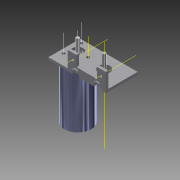
# Autodesk Inventor part: DC motor
Saved by Autodesk Inventor 2013 (Build 170138000, 138)
## iProperties
Created: 2013-01-03
Part Number: DC motor
Material: Generic
Document SubType Name: Modeling
Designer: Nico
Density: 1 g/cm^3
Author: Nico
Autodesk Inventor part; units mm, degrees
ref_plane "YZ Plane" through (0, 0, 0) normal (1, 0, 0) x (0, 1, 0)
ref_plane "XZ Plane" through (0, 0, 0) normal (0, 1, 0) x (-1, 0, 0)
ref_plane "XY Plane" through (0, 0, 0) normal (0, 0, 1) x (1, 0, 0)
sketch "Sketch1" plane through (0, 0, 0) normal (0, 0, 1) x (1, 0, 0)
  line L0 (0, 0) -> (90, 0)
  line L1 (90, 0) -> (90, 50)
  line L2 (90, 50) -> (0, 50)
  line L3 (0, 50) -> (0, 0)
  dimension "d0" = 50
  dimension "d1" = 90
  constraints: 8 end point, 2 parallel, 1 horizontal, 1 perpendicular
  measures "d0" distance of L2.end L0.start
  measures "d1" distance of L0.start L0.end
extrude "Extrusion1" add sketch "Sketch1" along normal blind 4
sketch "Sketch2" plane through (0, 0, 4) normal (0, 0, 1) x (1, 0, 0)
  line L0 (0, 0) -> (90, 0) projected
  line L1 (90, 0) -> (90, 50) projected
  line L2 (0, 50) -> (0, 0) projected
  line L3 (30, 0) -> (90, 0)
  line L4 (90, 0) -> (90, 4)
  line L5 (90, 4) -> (30, 4)
  line L6 (30, 4) -> (30, 0)
  dimension "d4" = 30
  dimension "d5" = 4
  constraints: 8 end point, 2 parallel, 2 point on line, 1 horizontal, 1 perpendicular
  measures "d4" distance between parallel lines of L2 L6
  measures "d5" distance between parallel lines of L0 L5
extrude "Extrusion2" add sketch "Sketch2" along normal blind 25
sketch "Sketch3" plane through (0, 0, 0) normal (0, -1, 0) x (1, 0, 0)
  line L0 (0, 0) -> (90, 0) projected
  line L1 (90, 0) -> (90, 29) projected
  line L2 (30, 29) -> (90, 29) projected
  line L3 (30, 4) -> (30, 29) projected
  line L4 (44, 29) -> (76, 29)
  line L5 (76, 29) -> (76, 12.5)
  line L6 (76, 12.5) -> (44, 12.5)
  line L7 (44, 12.5) -> (44, 29)
  arc A0 (49, 4) -> (37, 4) centre (43, 4) ccw
  line L8 (37, 0) -> (49, 0)
  line L9 (49, 0) -> (49, 4)
  line L10 (37, 4) -> (37, 0)
  line L11 (71, 0) -> (83, 0)
  line L12 (83, 0) -> (83, 4)
  line L13 (71, 4) -> (71, 0)
  arc A1 (83, 4) -> (71, 4) centre (77, 4) ccw
  dimension "d8" = 14
  dimension "d9" = 14
  dimension "d10" = 16.5
  dimension "d11" = 12
  dimension "d13" = 13
  dimension "d14" = 13
  constraints: 20 end point, 4 parallel, 4 point on circle, 3 horizontal, 3 perpendicular, 3 point on line, 2 centre point
  measures "d8" distance between parallel lines of L3 L7
  measures "d9" distance between parallel lines of L5 L1
  measures "d10" distance between parallel lines of L6 L2
  measures "d11" diameter of A0
  measures "d13" distance from line of A0.centre L3
  measures "d14" distance from line of A1.centre L1
extrude "Extrusion3" cut sketch "Sketch3" against normal blind 4
sketch "Sketch4" plane through (0, 0, 0) normal (0, -1, 0) x (1, 0, 0)
  line L0 (76, 29) -> (90, 29) projected
  line L1 (30, 29) -> (44, 29) projected
  line L2 (30, 4) -> (30, 29) projected
  point P0 (38, 19.75)
  point P1 (82, 19.75)
  dimension "d17" = 44
  dimension "d19" = 8
  dimension "d20" = 9.25
  dimension "d21" = 9.25
  measures "d17" distance of point (82, 19.75) point (38, 19.75)
  measures "d19" distance from line of L2 point (38, 19.75)
  measures "d20" distance from line of point (38, 19.75) L1
  measures "d21" distance from line of L0 point (82, 19.75)
hole "Hole1" at (38, 0, 19.75) at (82, 0, 19.75) direction (0, 1, 0) diameter 4.5 end through all
sketch "Sketch5" plane through (0, 0, 4) normal (0, 0, 1) x (1, 0, 0)
  line L0 (90, 50) -> (0, 50) projected
  line L1 (0, 50) -> (0, 0) projected
  circle A0 centre (15, 31) radius 8.5
  circle A1 centre (6.8969, 44.9883) radius 2.25
  circle A2 centre (31.1658, 31.0233) radius 2.25
  circle A3 centre (6.9373, 16.9883) radius 2.25
  dimension "d29" = 19
  dimension "d30" = 15
  dimension "d31" = 17
  dimension "d33" = 4.5
  dimension "d34" = 4.5
  dimension "d35" = 4.5
  constraints: 4 centre point, 1 coincident
  measures "d29" distance from line of A0.centre L0
  measures "d30" distance from line of L1 A0.centre
  measures "d31" diameter of A0
  measures "d33" diameter of A1
  measures "d34" diameter of A2
  measures "d35" diameter of A3
extrude "Extrusion4" cut sketch "Sketch5" against normal blind 4
sketch "Sketch6" plane through (0, 0, 0) normal (0, 0, -1) x (-1, 0, 0)
  circle A0 centre (-6.9373, 16.9883) radius 2.25 projected
  circle A1 centre (-6.8969, 44.9883) radius 2.25 projected
  circle A2 centre (-31.1658, 31.0233) radius 2.25 projected
  circle A3 centre (-6.8969, 44.9883) radius 4
  circle A4 centre (-31.1658, 31.0233) radius 4
  circle A5 centre (-6.9373, 16.9883) radius 4
  dimension "d38" = 8
  dimension "d40" = 8
  dimension "d41" = 8
  constraints: 3 centre point, 3 coincident
  measures "d38" diameter of A4
  measures "d40" diameter of A3
  measures "d41" diameter of A5
extrude "Extrusion5" add sketch "Sketch6" along normal blind 6.35
sketch "Sketch7" plane through (31.1658, 31.0233, -6.35) normal (0, 0, -1) x (-1, 0, 0)
  circle A0 centre (16.1658, 0) radius 21
  line L0 (31.1658, 18.9767) -> (31.1658, -31.0233) projected
  dimension "d44" = 42
  dimension "d47" = 15
  constraints: 1 centre point
  measures "d44" diameter of A0
  measures "d47" distance from line of L0 A0.centre
extrude "Extrusion6" add sketch "Sketch7" along normal blind 85
sketch "Sketch8" plane through (15, 31.0233, -6.35) normal (0, 0, 1) x (1, 0, 0)
  circle A0 centre (0, 0) radius 21 projected
  circle A1 centre (0, 0) radius 8.0116
  point P0 (-15, -31.0233)
  constraints: 1 centre point, 1 coincident
extrude "Extrusion7" add sketch "Sketch8" along normal blind 2 contours A1
sketch "Sketch9" plane through (15, 31.0233, -4.35) normal (0, 0, 1) x (1, 0, 0)
  circle A0 centre (0, 0) radius 8.0116 projected
  circle A1 centre (0, 0) radius 2.5
  point P0 (-15, -31.0233)
  dimension "d52" = 5
  constraints: 1 centre point, 1 coincident
  measures "d52" diameter of A1
extrude "Extrusion8" add sketch "Sketch9" along normal blind 27 contours A1
sketch "Sketch10" plane through (0, 0, 4) normal (0, 0, 1) x (1, 0, 0)
  line L0 (90, 4) -> (90, 50) projected
  line L1 (90, 50) -> (0, 50) projected
  circle A0 centre (60, 27.5) radius 9
  dimension "d56" = 22.5
  dimension "d57" = 30
  dimension "d58" = 18
  constraints: 1 centre point
  measures "d56" distance from line of A0.centre L1
  measures "d57" distance from line of L0 A0.centre
  measures "d58" diameter of A0
extrude "Extrusion9" cut sketch "Sketch10" against normal blind 4
sketch "Sketch11" plane through (0, 0, 0) normal (0, 0, -1) x (-1, 0, 0)
  circle A0 centre (-60, 27.5) radius 9 projected
  circle A1 centre (-60, 27.5) radius 10
  dimension "d61" = 20
  constraints: 1 centre point, 1 coincident
  measures "d61" diameter of A1
extrude "Extrusion10" add sketch "Sketch11" along normal blind 14
sketch "Sketch12" plane through (60, 27.5, -14) normal (0, 0, -1) x (-1, 0, 0)
  circle A0 centre (0, 0) radius 10 projected
  point P0 (60, -27.5)
extrude "Extrusion11" add sketch "Sketch12" against normal blind 3
fillet "Fillet1" radius 2 1 edges at (70, 27.5, -14)
sketch "Sketch13" plane through (0, 0, 4) normal (0, 0, 1) x (1, 0, 0)
  circle A0 centre (60, 27.5) radius 9 projected
  circle A1 centre (60, 27.5) radius 2.5
  dimension "d68" = 5
  constraints: 1 centre point, 1 coincident
  measures "d68" diameter of A1
extrude "Extrusion12" add sketch "Sketch13" along normal blind 22 contours A1
body "Solid1"
